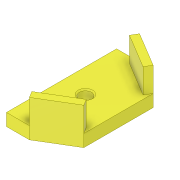
# Autodesk Inventor part: 30_Cube_Z_Focus_Drylin_NEMA_slide_part1
Saved by Autodesk Inventor 2019.4 (Build 234330000, 330)
## iProperties
Created: 2021-05-05
Part Number: 30_Cube_Z_Focus_Drylin_NEMA_slide_part1
Material: Generic
Document SubType Name: Modeling
Designer: diederichbenedict
Density: 1 g/cm^3
Appearance: Smooth - Yellow
Author: diederichbenedict
Autodesk Inventor part; units mm, degrees
ref_plane "YZ Plane" through (0, 0, 0) normal (1, 0, 0) x (0, 1, 0)
ref_plane "XZ Plane" through (0, 0, 0) normal (0, 1, 0) x (-1, 0, 0)
ref_plane "XY Plane" through (0, 0, 0) normal (0, 0, 1) x (1, 0, 0)
sketch "Sketch1" plane through (0, 0, 0) normal (0, 1, 0) x (-1, 0, 0)
  line L0 (-13.5, -18.4952) -> (9.75, -18.4952)
  line L1 (9.75, -18.4952) -> (9.75, 18.4952)
  line L2 (9.75, 18.4952) -> (-13.5, 18.4952)
  line L3 (-13.5, 18.4952) -> (-13.5, -18.4952)
  circle A0 centre (-7.5, 0) radius 4
  circle A1 centre (3.75, -6.4952) radius 4
  circle A2 centre (3.75, 6.4952) radius 4
  circle A3 centre (0, 0) radius 7.5 construction
  circle A4 centre (0, 0) radius 2.5
  dimension "d11" = 15
  dimension "d2" = 8
  dimension "d6" = 360
  dimension "d8" = 6
  dimension "d9" = 6
  dimension "d1" = 12
  dimension "d13" = 12
  dimension "d35" = 5
  constraints: 8 end point, 4 centre point, 2 parallel, 1 coincident, 1 horizontal, 1 horizontal alignment, 1 perpendicular, 9 other
  measures "d2" diameter of A0
  measures "d8" distance from line of A2.centre L1
  measures "d9" distance from line of L3 A0.centre
  measures "d1" distance from line of L2 A2.centre
  measures "d13" distance from line of L0 A1.centre
  measures "d35" diameter of A4
extrude "Extrusion1" add sketch "Sketch1" along normal blind 4
sketch "Sketch2" plane through (0, 4, 0) normal (0, 1, 0) x (1, 0, 0)
  circle A0 centre (-3.75, -6.4952) radius 4 projected
  circle A1 centre (-3.75, 6.4952) radius 4 projected
  circle A2 centre (7.5, 0) radius 4 projected
  line L0 (13.5, 18.4952) -> (-9.75, 18.4952) projected
  line L1 (-9.75, 18.4952) -> (-9.75, -18.4952) projected
  line L2 (-9.75, -18.4952) -> (13.5, -18.4952) projected
  line L3 (13.5, -18.4952) -> (13.5, 18.4952) projected
  circle A3 centre (0, 0) radius 2.5
  dimension "d16" = 5
  constraints: 1 centre point, 1 coincident
  measures "d16" diameter of A3
extrude "Extrusion2" add sketch "Sketch2" along normal blind 1 contours A0 | A1 | A2 | L3 L2 L1 L0
sketch "Sketch3" plane through (0, 0, 0) normal (0, -1, 0) x (1, 0, 0)
  circle A0 centre (-3.75, 6.4952) radius 4 projected
  circle A1 centre (-3.75, -6.4952) radius 4 projected
  circle A2 centre (7.5, 0) radius 4 projected
  line L0 (13.5, -18.4952) -> (-9.75, -18.4952) projected
  line L1 (13.5, 18.4952) -> (13.5, -18.4952) projected
  line L2 (-9.75, 18.4952) -> (13.5, 18.4952) projected
  line L3 (-9.75, -18.4952) -> (-9.75, 18.4952) construction
  line L4 (-1.5, 18.4952) -> (13.5, 9.4952)
  line L5 (13.5, 18.4952) -> (13.5, -18.4952) projected
  line L6 (13.5, -9.4952) -> (-1.5, -18.4952)
  point P0 (0, 0)
  dimension "d19" = 9
  dimension "d20" = 9
  dimension "d21" = 15
  dimension "d22" = 15
  constraints: 4 end point, 4 point on line
  measures "d19" distance from line of L2 L4.end
  measures "d20" distance from line of L0 L6.start
  measures "d21" distance from line of L6.end L1
  measures "d22" distance from line of L1 L4.start
extrude "Extrusion3" cut sketch "Sketch3" against normal through all contours L4 L2 L1 | L0 L6 L1
sketch "Sketch5" plane through (0, 0, 0) normal (0, -1, 0) x (1, 0, 0)
  line L0 (13.5, 9.4952) -> (-1.5, 18.4952) projected
  line L1 (-9.75, 18.4952) -> (-1.5, 18.4952) projected
  line L2 (-9.75, -18.4952) -> (-9.75, 18.4952) projected
  line L3 (-1.5, -18.4952) -> (-9.75, -18.4952) projected
  line L4 (-1.5, -18.4952) -> (13.5, -9.4952) projected
  line L5 (13.5, 9.4952) -> (13.5, -9.4952) projected
  circle A0 centre (-3.75, 6.4952) radius 4 projected
  circle A1 centre (-3.75, -6.4952) radius 4 projected
  circle A2 centre (7.5, 0) radius 4 projected
  line L6 (17.5, -11.76) -> (-0.3921, -22.4952)
  line L7 (-0.3921, -22.4952) -> (-13.75, -22.4952)
  line L8 (-13.75, -22.4952) -> (-13.75, 22.4952)
  line L9 (-13.75, 22.4952) -> (-0.3921, 22.4952)
  line L10 (-0.3921, 22.4952) -> (17.5, 11.76)
  line L11 (17.5, 11.76) -> (17.5, -11.76)
  line L12 (13.5, -9.4952) -> (13.5, -14.16)
  line L13 (13.5, 3.4118) -> (13.5, 14.16)
  line L14 (-1.5, -18.4952) -> (-9.75, -18.4952) projected
  line L15 (-9.75, -18.4952) -> (-9.75, -22.4952)
  line L16 (-9.75, 18.4952) -> (-1.5, 18.4952) projected
  line L17 (-9.75, 18.4952) -> (-9.75, 22.4952)
  line L18 (-1.5, -18.4952) -> (13.5, -9.4952) projected
  line L19 (13.5, -9.4952) -> (-1.5, -18.4952)
  line L20 (-1.5, -18.4952) -> (-9.75, -18.4952)
  line L21 (-9.75, -18.4952) -> (-9.75, 18.4952) projected
  line L22 (-9.75, 18.4952) -> (-1.5, 18.4952)
  line L23 (13.5, 9.4952) -> (-1.5, 18.4952) projected
  line L24 (13.5, 9.4952) -> (-1.5, 18.4952)
  line L25 (13.5, -9.4952) -> (13.5, 3.4118)
  point P0 (0, 0)
  dimension "d27" = 4
  constraints: 30 end point, 6 point on line, 4 collinear, 2 perpendicular, 2 vertical, 5 other
  measures "d27" distance between parallel lines of L4 L6
extrude "Extrusion5" add sketch "Sketch5" against normal up to surface (5 mm away) contours L0 L1 L17 L9 L10 L13 | L12 L6 L7 L15 L3 L4
sketch "Sketch6" plane through (0, 5, 0) normal (0, 1, 0) x (1, 0, 0)
  line L0 (13.5, -14.16) -> (13.5, 14.16) projected
  line L1 (-0.3921, 22.4952) -> (13.5, 14.16) projected
  line L2 (-9.75, 22.4952) -> (-0.3921, 22.4952) projected
  line L3 (-9.75, -22.4952) -> (-9.75, 22.4952) projected
  line L4 (-0.3921, -22.4952) -> (-9.75, -22.4952) projected
  line L5 (13.5, -14.16) -> (-0.3921, -22.4952) projected
  line L6 (13.5, 14.16) -> (-0.3921, 22.4952)
  line L7 (-0.3921, 22.4952) -> (-1.9356, 19.9227)
  line L8 (-1.9356, 19.9227) -> (11.9565, 11.5875)
  line L9 (11.9565, 11.5875) -> (13.5, 14.16)
  line L10 (13.5, -14.16) -> (13.5, 14.16) projected
  line L11 (13.5, -14.16) -> (-0.3921, -22.4952)
  line L12 (-0.3921, -22.4952) -> (-1.9356, -19.9227)
  line L13 (-1.9356, -19.9227) -> (11.9565, -11.5875)
  line L14 (11.9565, -11.5875) -> (13.5, -14.16)
  point P0 (0, 0)
  dimension "d30" = 3
  dimension "d31" = 3
  constraints: 16 end point, 5 equal length, 2 perpendicular
  measures "d30" distance of L7.end L1.start
  measures "d31" distance of L4.start L12.end
extrude "Extrusion6" add sketch "Sketch6" along normal blind 10 contours L5 L12 L13 L14 | L9 L8 L7 L1
chamfer "Chamfer1" distance 0.5 angle 45 5 edges at (2.5, 0, 0) (-2.5, 5, 0) (0.25, 0, 6.4952) (11.5, 0, 0) (0.25, 0, -6.4952)
equation "\"d13\" = d1"
body "Solid1"
